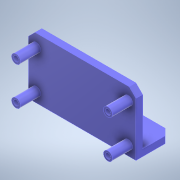
# Autodesk Inventor part: ultrasonic and headlight mount
Saved by Autodesk Inventor 2022.6 (Build 266554000, 554)
## iProperties
Created: 2024-06-19
Part Number: ultrasonic and headlight mount
Material: Generic
Document SubType Name: Modeling
Designer: david
Density: 1 g/cm^3
Appearance: Smooth - Dark Forest Green
Description: Mount for Ultrasonic sensor
Mass: 6.22198 g
Surface Area: 48.5677 cm^2
Volume: 6.22198 cm^3
Author: david
Autodesk Inventor part; units mm, degrees
ref_plane "YZ Plane" through (0, 0, 0) normal (1, 0, 0) x (0, 1, 0)
ref_plane "XZ Plane" through (0, 0, 0) normal (0, 1, 0) x (-1, 0, 0)
ref_plane "XY Plane" through (0, 0, 0) normal (0, 0, 1) x (1, 0, 0)
sketch "Sketch1" plane through (0, 0, 0) normal (0, 0, 1) x (1, 0, 0)
  line L0 (-22, 22) -> (22, 22) construction
  line L1 (22, 22) -> (22, 2) construction
  line L2 (22, 2) -> (-22, 2) construction
  line L3 (-22, 2) -> (-22, 22) construction
  line L4 (-22, 22) -> (22, 2) construction
  line L5 (22, 22) -> (-22, 2) construction
  line L6 (24, 24) -> (-24, 24)
  line L7 (-24, 24) -> (-24, 0)
  line L8 (-24, 0) -> (24, 0)
  line L9 (24, 0) -> (24, 24)
  line L10 (10, 24) -> (-10, 24)
  line L11 (-10, 24) -> (-10, 56)
  line L12 (-10, 56) -> (10, 56)
  line L13 (10, 56) -> (10, 24)
  line L14 (0, -11.2) -> (0, 67.2) projected
  point P0 (0, 12)
  point P1 (0, 12)
  point P2 (0, 0)
  point P3 (0, 12)
  dimension "d0" = 20
  dimension "d1" = 44
  dimension "d2" = 2
  dimension "d53" = 32
  dimension "d54" = 20
  constraints: 28 end point, 6 parallel, 5 midpoint, 3 perpendicular, 2 horizontal, 1 point on line, 1 vertical alignment, 4 other
  measures "d0" distance of L0.end L1.end
  measures "d1" distance of L1.end L2.end
  measures "d2" distance between parallel lines of L0 L6
  measures "d53" distance of L10.end L11.end
  measures "d54" distance of L11.end L12.end
extrude "Extrusion1" add sketch "Sketch1" against normal blind 3 contours L9 L8 L14 L6 | L14 L8 L7 L6
sketch "Sketch2" plane through (-24, 0, 0) normal (0, -1, 0) x (1, 0, 0)
  line L0 (48, 0) -> (0, 0) projected
  line L1 (48, 0) -> (0, 0)
  line L2 (0, 0) -> (0, -16)
  line L3 (0, -16) -> (48, -16)
  line L4 (48, -16) -> (48, 0)
  point P0 (24, 0)
  point P1 (0, -3)
  point P2 (0, 0)
  dimension "d5" = 16
  constraints: 8 end point, 2 parallel, 1 horizontal, 1 perpendicular, 1 vertical alignment
  measures "d5" distance between parallel lines of L0 L3
extrude "Extrusion2" add sketch "Sketch2" along normal blind 3
sketch "Sketch3" plane through (0, 0, 0) normal (0, 0, 1) x (1, 0, 0)
  line L0 (-24, 24) -> (-24, -3) projected
  line L1 (24, -3) -> (-24, -3) projected
  line L2 (24, -3) -> (24, 24) projected
  line L3 (24, 24) -> (-24, 24) projected
  line L4 (-20.5, 18.5) -> (20.5, 18.5) construction
  line L5 (20.5, 18.5) -> (20.5, 1.5) construction
  line L6 (20.5, 1.5) -> (-20.5, 1.5) construction
  line L7 (-20.5, 1.5) -> (-20.5, 18.5) construction
  line L8 (-20.5, 18.5) -> (20.5, 1.5) construction
  line L9 (20.5, 18.5) -> (-20.5, 1.5) construction
  line L10 (0, 29.4) -> (0, -8.4) projected
  point P0 (0, 10)
  dimension "d73" = 41
  dimension "d74" = 17
  constraints: 12 end point, 4 coincident, 2 parallel, 1 horizontal, 1 midpoint, 1 perpendicular, 1 point on line
  measures "d73" distance of L5.end L6.end
  measures "d74" distance of L6.end L4.start
hole "Hole1" at (-20.5, 18.5, 0) at (20.5, 18.5, 0) at (20.5, 1.5, 0) at (-20.5, 1.5, 0) direction (0, 0, -1) diameter 2.4 end through all
sketch "Sketch4" plane through (0, 0, 0) normal (1, 0, 0) x (0, 1, 0)
  line L0 (0, -3) -> (24, -3) projected
  line L1 (23.7, -3) -> (0, -15)
  line L2 (24, -3) -> (0, -3) projected
  line L3 (24, -3) -> (0, -3) projected
  line L4 (0, -16) -> (-3, -16) projected
  line L5 (-3, 0) -> (24, 0) projected
  line L6 (0, -3) -> (0, -16) projected
  line L7 (-3, -16) -> (-3, 0) projected
  line L8 (24, 0) -> (24, -3) projected
  point P0 (3, -3)
  dimension "d21" = 12
  dimension "d22" = 23.7
  constraints: 2 end point, 2 point on line
  measures "d21" distance of L1.end L0.start
  measures "d22" distance of L0.start L1.start
extrude "Rib1" add sketch "Sketch4" along normal mid plane 3 rib yes fills toward (11.8274, -8.9554) open curves L1
chamfer "Chamfer1" [suppressed]
sketch "Sketch5" plane through (-24, 0, 0) normal (0, 1, 0) x (1, 0, 0)
  line L0 (0, 16) -> (48, 16) projected
  line L1 (9, 9.5) -> (39, 9.5)
  line L2 (0, 3) -> (48, 3) projected
  line L3 (48, 0) -> (48, 3) projected
  line L4 (48, 3) -> (48, 16)
  line L5 (0, 16) -> (48, 16) projected
  line L6 (48, 3) -> (48, 16)
  line L7 (48, 0) -> (48, 16) projected
  line L8 (25.5, 3) -> (22.5, 3) projected
  line L9 (24, 3) -> (24, 16)
  line L10 (48, 16) -> (48, 3) projected
  line L11 (0, 3) -> (22.5, 3) projected
  line L12 (0, 0) -> (0, 3) projected
  line L13 (48, 0) -> (0, 0) projected
  line L14 (48, 3) -> (48, 0) projected
  line L15 (0, 3) -> (0, 16) projected
  line L16 (22.5, 3) -> (22.5, 15) projected
  line L17 (22.5, 15) -> (25.5, 15) projected
  line L18 (25.5, 15) -> (25.5, 3) projected
  line L19 (25.5, 3) -> (48, 3) projected
  point P0 (24, 0)
  point P1 (24, 9.5)
  point P2 (24, 9.5)
  dimension "d32" = 30
  constraints: 8 end point, 5 midpoint, 2 perpendicular, 1 collinear, 1 horizontal, 1 horizontal alignment, 1 vertical alignment
  measures "d32" distance of L1.end L1.start
hole "Hole2" at (15, 0, -9.5) at (-15, 0, -9.5) direction (0, -1, 0) diameter 3.4 depth 6
chamfer "Chamfer2" distance 3 angle 45 4 edges at (24, -1.5, -16) (-24, -1.5, -16) (-24, 24, -1.5) (24, 24, -1.5)
sketch "Sketch6" plane through (0, 0, 0) normal (0, 0, 1) x (1, 0, 0)
  circle A0 centre (-20.5, 18.5) radius 2
  circle A1 centre (20.5, 18.5) radius 2
  circle A2 centre (20.5, 1.5) radius 2
  circle A3 centre (-20.5, 1.5) radius 2
  circle A4 centre (-20.5, 18.5) radius 1.2 projected
  circle A5 centre (-20.5, 1.5) radius 1.2 projected
  circle A6 centre (20.5, 18.5) radius 1.2 projected
  circle A7 centre (20.5, 1.5) radius 1.2 projected
  point P0 (0, 0)
  point P1 (-20.5, 20.5)
  point P2 (20.5, 20.5)
  point P3 (20.5, 3.5)
  point P4 (-20.5, 3.5)
  dimension "d46" = 4
  dimension "d47" = 4
  dimension "d49" = 4
  dimension "d50" = 4
  constraints: 4 centre point, 4 coincident
  measures "d46" diameter of A0
  measures "d47" diameter of A1
  measures "d49" diameter of A2
  measures "d50" diameter of A3
extrude "Extrusion3" add sketch "Sketch6" along normal blind 9
sketch "Sketch7" plane through (0, 0, 0) normal (0, 0, 1) x (1, 0, 0)
  circle A0 centre (20.5, 1.5) radius 2 projected
  circle A1 centre (-20.5, 1.5) radius 2 projected
  circle A2 centre (20.5, 18.5) radius 2 projected
  circle A3 centre (-20.5, 18.5) radius 2 projected
  line L0 (21, 24) -> (24, 21) projected
  line L1 (21, 24) -> (-21, 24) projected
  line L2 (-24, 21) -> (-21, 24) projected
  line L3 (-24, 21) -> (-24, -3) projected
  line L4 (24, -3) -> (-24, -3) projected
  line L5 (24, -3) -> (24, 21) projected
  circle A4 centre (0, 48) radius 4.25
  line L6 (0, -14.8) -> (0, 67.8) projected
  point P0 (0, 0)
  dimension "d55" = 8.5
  dimension "d57" = 24
  constraints: 1 centre point, 1 point on line
  measures "d55" diameter of A4
  measures "d57" distance from line of L1 A4.centre
extrude "Extrusion4" [suppressed]
sketch "Sketch9" plane through (0, 0, 0) normal (0, 0, 1) x (1, 0, 0)
  circle A0 centre (20.5, 1.5) radius 2 projected
  circle A1 centre (-20.5, 1.5) radius 2 projected
  circle A2 centre (20.5, 18.5) radius 2 projected
  circle A3 centre (-20.5, 18.5) radius 2 projected
  line L0 (21, 24) -> (-21, 24) projected
  line L1 (-24, 21) -> (-21, 24) projected
  line L2 (-24, 21) -> (-24, -3) projected
  line L3 (24, -3) -> (-24, -3) projected
  line L4 (24, -3) -> (24, 21) projected
  line L5 (21, 24) -> (24, 21) projected
  line L6 (-10, 24) -> (-21, 24) projected
  line L7 (10, 24) -> (10, 56) projected
  line L8 (-10, 24) -> (10, 24)
  point P0 (0, 0)
  point P1 (10, 53)
  constraints: 2 end point, 1 horizontal
feature "Bend Part1" [suppressed]
sketch "Sketch10" plane through (10, 24, 0) normal (1, 0, 0) x (0, 0, -1)
  line L0 (0, 0) -> (0, 32) projected
  line L1 (0, 0) -> (3, 0) projected
  line L2 (3, 32) -> (3, 0) projected
  line L3 (3, 29) -> (3, 32) projected
  line L4 (3, 32) -> (0, 32) projected
  line L5 (0, 32) -> (0, 29) projected
  line L6 (0, 29) -> (3, 29) projected
  line L7 (0, 32) -> (1, 32)
  line L8 (1, 32) -> (1, 2)
  line L9 (1, 2) -> (0, 2)
  line L10 (0, 2) -> (0, 32)
  line L11 (0, 32) -> (3, 32) projected
  point P0 (0, -24)
  point P1 (0, 2)
  dimension "d66" = 1
  dimension "d67" = 30
  constraints: 8 end point, 2 parallel, 1 horizontal, 1 perpendicular
  measures "d66" distance of L8.end L9.end
  measures "d67" distance of L7.end L8.end
extrude "Extrusion6" [suppressed]
chamfer "Chamfer3" [suppressed]
sketch "Sketch11" plane through (0, 0, 0) normal (0, 0, 1) x (1, 0, 0)
  line L0 (2.5, 2) -> (2.5, 19.75) projected
  circle A0 centre (-20.5, 18.5) radius 2 projected
  circle A1 centre (20.5, 18.5) radius 2 projected
  circle A2 centre (-20.5, 1.5) radius 2 projected
  circle A3 centre (20.5, 1.5) radius 2 projected
  line L1 (21, 24) -> (-21, 24) projected
  line L2 (-24, 21) -> (-21, 24) projected
  line L3 (-24, 21) -> (-24, -3) projected
  line L4 (24, -3) -> (-24, -3) projected
  line L5 (24, -3) -> (24, 21) projected
  line L6 (21, 24) -> (24, 21) projected
  line L7 (-5, 23.7) -> (5, 23.7)
  line L8 (5, 23.7) -> (5, 26.7)
  line L9 (5, 26.7) -> (-5, 26.7)
  line L10 (-5, 26.7) -> (-5, 23.7)
  line L11 (5, 26.7) -> (-5, 23.7) construction
  line L12 (5, 23.7) -> (-5, 26.7) construction
  line L13 (0, 67.8) -> (0, -14.8) construction
  point P0 (0, 0)
  point P1 (0, 25.2)
  point P2 (0, 25.2)
  dimension "d77" = 10
  dimension "d78" = 3
  constraints: 12 end point, 2 midpoint, 2 parallel, 1 horizontal, 1 perpendicular, 1 point on line
  measures "d77" distance of L8.end L9.end
  measures "d78" distance of L7.end L8.end
extrude "Extrusion7" [suppressed]
sketch "Sketch12" plane through (0, 0, -3) normal (0, 0, -1) x (-1, 0, 0)
  circle A0 centre (20.5, 1.5) radius 1.2 projected
  circle A1 centre (-20.5, 18.5) radius 1.2 projected
  circle A2 centre (20.5, 18.5) radius 1.2 projected
  circle A3 centre (-20.5, 1.5) radius 1.2 projected
  line L0 (1.5, 0) -> (24, 0) projected
  line L1 (24, 0) -> (24, 21) projected
  line L2 (21, 24) -> (24, 21) projected
  line L3 (21, 24) -> (-21, 24) projected
  line L4 (-24, 21) -> (-21, 24) projected
  line L5 (-24, 21) -> (-24, 0) projected
  line L6 (-24, 0) -> (-1.5, 0) projected
  line L7 (-21, 24) -> (-10, 24) projected
  line L8 (-10, 24) -> (-5, 24)
  line L9 (-5, 24) -> (-5, 28)
  line L10 (-5, 28) -> (-10, 28)
  line L11 (-10, 28) -> (-10, 24)
  line L12 (10, 24) -> (5, 24)
  line L13 (5, 24) -> (5, 28)
  line L14 (5, 28) -> (10, 28)
  line L15 (10, 28) -> (10, 24)
  line L16 (5, 26.7) -> (5, 23.7) projected
  line L17 (-5, 23.7) -> (-5, 26.7) projected
  line L18 (1.5, 23.7) -> (1.5, 0) projected
  line L19 (-1.5, 0) -> (-1.5, 23.7) projected
  line L20 (-1.5, 23.7) -> (1.5, 23.7) projected
  point P0 (0, 0)
  dimension "d81" = 4
  dimension "d82" = 4
  constraints: 16 end point, 4 parallel, 2 collinear, 2 horizontal, 2 perpendicular
  measures "d81" distance of L9.end L8.end
  measures "d82" distance of L12.end L13.end
extrude "Extrusion8" [suppressed]
chamfer "Chamfer4" distance 2 angle 45 4 edges at (1.5, 11.85, -3) (-1.5, 11.85, -3) (-1.5, 0, -9) (1.5, 0, -9)
equation "\"d46\" = d50"
equation "\"d47\" = d50"
equation "\"d49\" = d50"
body "Solid1"
